Autodesk Fusion 360 part; units mm, degrees
(part 2 of 2)
sketch "Sketch43" plane through (0, 10, 0) normal (0, 1, 0) x (-1, 0, 0)
  line L0 (-47.7, 203) -> (-47.7, 218)
  line L1 (-47.7, 218) -> (-127.2, 218)
  line L2 (-127.2, 218) -> (-127.2, -25)
  line L3 (-127.2, -25) -> (-46.7, -25)
  line L4 (-46.7, -25) -> (-46.7, -10)
  line L5 (-46.7, -10) -> (15, -10)
  line L6 (15, -10) -> (15, -15)
  line L7 (15, -15) -> (30, -15)
  line L8 (30, -15) -> (30, 198)
  line L9 (30, 198) -> (17.475, 208)
  line L10 (17.475, 208) -> (15, 208)
  line L11 (15, 208) -> (15, 203)
  line L12 (15, 203) -> (-47.7, 203)
  circle A0 centre (-63.325, 91) radius 4
  circle A1 centre (-105.075, 102) radius 4
  line L13 (15, 208) -> (30, 208)
  line L14 (30, 208) -> (30, 203)
  line L15 (30, 203) -> (15, 203)
  line L16 (15, 203) -> (15, 208)
  line L17 (30, 203) -> (-47.7, 203)
  line L18 (-47.7, 203) -> (-47.7, 198)
  line L19 (-47.7, 198) -> (30, 198)
  line L20 (30, 198) -> (30, 203)
  line L21 (30, -15) -> (15, -15)
  line L22 (15, -15) -> (15, -10)
  line L23 (15, -10) -> (30, -10)
  line L24 (30, -10) -> (30, -15)
  line L25 (-46.7, -10) -> (30, -10)
  line L26 (30, -10) -> (30, -5)
  line L27 (30, -5) -> (-46.7, -5)
  line L28 (-46.7, -5) -> (-46.7, -10)
  line L29 (15, -10) -> (-46.7, -10)
  line L30 (-46.7, -10) -> (-46.7, -5)
  line L31 (-46.7, -5) -> (15, -5)
  line L32 (15, -5) -> (15, -10)
  dimension "d251" = 15
  dimension "d252" = 5
  dimension "d253" = 5
  dimension "d254" = 15
  dimension "d255" = 5
  dimension "d256" = 5
  constraint horizontal L13
  constraint vertical L14
  constraint horizontal L15
  constraint vertical L16
  constraint coincident L10.end L11.start
  constraint horizontal L17
  constraint vertical L18
  constraint horizontal L19
  constraint vertical L20
  constraint horizontal L21
  constraint vertical L22
  constraint horizontal L23
  constraint vertical L24
  constraint coincident L7.end L8.start
  constraint horizontal L25
  constraint vertical L26
  constraint horizontal L27
  constraint vertical L28
  constraint coincident L4.end L5.start
  constraint horizontal L29
  constraint vertical L30
  constraint horizontal L31
  constraint vertical L32
  measures "d251" distance of L10.end L13.end
  measures "d252" distance of L10.end L11.end
  measures "d253" distance of L14.end L8.end
  measures "d254" distance of L7.end L6.end
  measures "d255" distance of L7.end L23.end
  measures "d256" distance of L4.end L27.end
extrude "Extrude87" cut sketch "Sketch43" against normal blind 5 contours L5 L25 L27 L28 L29 L30 L31 L32 bodies 1
extrude "Extrude88" cut 1 faces at (-25, 8.3333, -15) along direction (0, 0, 1) blind 5 on bodies 1 bodies 1
sketch "Sketch44" plane through (0, 10, 0) normal (0, 1, 0) x (-1, 0, 0)
  line L0 (15, -10) -> (30, -10)
  line L1 (30, -10) -> (30, 198)
  line L2 (30, 198) -> (17.475, 208)
  line L3 (17.475, 208) -> (15, 208)
  line L4 (15, 208) -> (15, 203)
  line L5 (15, 203) -> (-47.7, 203)
  line L6 (-47.7, 203) -> (-47.7, 218)
  line L7 (-47.7, 218) -> (-127.2, 218)
  line L8 (-127.2, 218) -> (-127.2, -25)
  line L9 (-127.2, -25) -> (-46.7, -25)
  line L10 (-46.7, -25) -> (-46.7, -5)
  line L11 (-46.7, -5) -> (15, -5)
  line L12 (15, -5) -> (15, -10)
  circle A0 centre (-63.325, 91) radius 4
  circle A1 centre (-105.075, 102) radius 4
  line L13 (15, 208) -> (30, 208)
  line L14 (30, 208) -> (30, 198)
  line L15 (30, 198) -> (15, 198)
  line L16 (15, 198) -> (15, 208)
  line L17 (15, 203) -> (30, 203)
  line L18 (30, 203) -> (30, 198)
  line L19 (30, 198) -> (15, 198)
  line L20 (15, 198) -> (15, 203)
  line L21 (17.475, 208) -> (30, 198)
  constraint horizontal L13
  constraint vertical L14
  constraint horizontal L15
  constraint vertical L16
  constraint coincident L1.end L2.start
  constraint coincident L3.end L4.start
  constraint horizontal L17
  constraint vertical L18
  constraint horizontal L19
  constraint vertical L20
  constraint coincident L4.end L5.start
  constraint coincident L2.end L3.start
extrude "Extrude89" cut 1 faces at (5.9, 8.3333, 203) along direction (0, 0, -1) blind 5 on bodies 1 bodies 1
sketch "Sketch45" plane through (0, 10, 0) normal (0, 1, 0) x (-1, 0, 0)
  line L0 (30, 198) -> (15, 198)
  line L1 (17.475, 208) -> (17.475, 198)
  line L2 (30, 198) -> (15, 198)
  line L3 (15, 198) -> (15, 193)
  line L4 (15, 193) -> (30, 193)
  line L5 (30, 193) -> (30, 198)
  line L6 (17.475, 203) -> (30, 193)
  point P0 (17.475, 208)
  dimension "d263" = 5
  constraint coincident P0 L1.start
  constraint coincident L0 L1.end
  constraint perpendicular L0 L1
  constraint horizontal L2
  constraint vertical L3
  constraint horizontal L4
  constraint vertical L5
  constraint coincident L0.start L2.start
  constraint midpoint L1 L6.start
  measures "d263" distance of L0.start L4.end
extrude "Extrude90" cut sketch "Sketch44" sketch "Sketch45" against normal blind 5 contours L2 L3 L4 L13 L16 L17 L21 of sketch 2 contours L0 L2 L5 L6 bodies 1
sketch "Sketch46" plane through (0, 10, 0) normal (0, 1, 0) x (-1, 0, 0)
  line L0 (23.7375, 203) -> (15, 203)
  line L1 (15, 203) -> (15, 198)
  line L2 (15, 198) -> (-47.7, 198)
  line L3 (-47.7, 198) -> (-47.7, 218)
  line L4 (-47.7, 218) -> (-127.2, 218)
  line L5 (-127.2, 218) -> (-127.2, -25)
  line L6 (-127.2, -25) -> (-46.7, -25)
  line L7 (-46.7, -25) -> (-46.7, -5)
  line L8 (-46.7, -5) -> (15, -5)
  line L9 (15, -5) -> (15, -10)
  line L10 (15, -10) -> (30, -10)
  line L11 (30, -10) -> (30, 193)
  line L12 (30, 193) -> (23.7375, 198)
  line L13 (23.7375, 198) -> (30, 198)
  line L14 (30, 198) -> (23.7375, 203)
  circle A0 centre (-105.075, 102) radius 4
  circle A1 centre (-63.325, 91) radius 4
  line L15 (15, 203) -> (17.475, 203)
  line L16 (17.475, 203) -> (17.475, 198)
  line L17 (17.475, 198) -> (15, 198)
  line L18 (15, 198) -> (15, 203)
  line L19 (23.7375, 198) -> (17.475, 203)
  dimension "d266" = 2.475
  constraint horizontal L15
  constraint vertical L16
  constraint horizontal L17
  constraint vertical L18
  constraint coincident L0.end L1.start
  constraint coincident L12.end L13.start
  measures "d266" distance of L0.end L15.end
extrude "Extrude91" cut sketch "Sketch46" against normal blind 5 contours L0 L13 L14 L19 bodies 1
sketch "Sketch47" plane through (0, 10, 0) normal (0, 1, 0) x (-1, 0, 0)
  line L0 (30, 193) -> (17.475, 203)
  line L1 (17.475, 203) -> (15, 203)
  line L2 (15, 203) -> (15, 198)
  line L3 (15, 198) -> (-47.7, 198)
  line L4 (-47.7, 198) -> (-47.7, 218)
  line L5 (-47.7, 218) -> (-127.2, 218)
  line L6 (-127.2, 218) -> (-127.2, -25)
  line L7 (-127.2, -25) -> (-46.7, -25)
  line L8 (-46.7, -25) -> (-46.7, -5)
  line L9 (-46.7, -5) -> (15, -5)
  line L10 (15, -5) -> (15, -10)
  line L11 (15, -10) -> (30, -10)
  line L12 (30, -10) -> (30, 193)
  circle A0 centre (-105.075, 102) radius 4
  circle A1 centre (-63.325, 91) radius 4
  line L13 (30, -10) -> (15, -10)
  line L14 (15, -10) -> (15, 13.5)
  line L15 (15, 13.5) -> (30, 13.5)
  line L16 (30, 13.5) -> (30, -10)
  line L17 (30, 13.5) -> (30, 193)
  line L18 (30, 193, 0) -> (30, 193, -5)
  line L19 (30, 193, -5) -> (30, 13.5, -5)
  line L20 (30, 13.5, -5) -> (30, 13.5, 0)
  point P0 (30, 193)
  dimension "d269" = 23.5
  constraint horizontal L13
  constraint vertical L14
  constraint horizontal L15
  constraint vertical L16
  constraint coincident L11.end L12.start
  constraint vertical L17
  constraint coincident P0 L0.start
  measures "d269" distance of L11.end L15.end
extrude "Extrude92" add sketch "Sketch47" along normal blind 10 contours L12 L17 L18 L19 L20 in plane through (-30, 10, 0) normal (-1, 0, 0) bodies 1
sketch "Sketch48" plane through (0, 0, 0) normal (0, 0, 1) x (1, 0, 0)
  point P0 (-15, 10)
extrude "Extrude93" add 1 faces at (-15, 8.3333, 201.3333) along direction (1, 0, 0) blind 62.7 on bodies 1 bodies 1
sketch "Sketch49" plane through (46.7, 0, 0) normal (-1, 0, 0) x (0, 0, 1)
  line L0 (-5, 10) -> (-25, 10)
  line L1 (-25, 10) -> (-25, -20)
  line L2 (-25, -20) -> (-5.4, -20)
  line L3 (-5.4, -20) -> (-5.4, 0)
  line L4 (-5.4, 0) -> (-5, 0)
  line L5 (-5, 0) -> (-5, 10)
  line L6 (-5, 10) -> (-25, 10)
  line L7 (-25, 10) -> (-25, 0)
  line L8 (-25, 0) -> (-5, 0)
  line L9 (-5, 0) -> (-5, 10)
  line L10 (-5, 10) -> (-17.5, 10)
  line L11 (-17.5, 10) -> (-17.5, 0)
  line L12 (-17.5, 0) -> (-5, 0)
  line L13 (-5, 0) -> (-5, 10)
  line L14 (-17.5, 10) -> (-25, 0)
  dimension "d274" = 20
  dimension "d275" = 10
  dimension "d276" = 12.5
  constraint horizontal L6
  constraint vertical L7
  constraint horizontal L8
  constraint vertical L9
  constraint coincident L0.start L5.end
  constraint horizontal L10
  constraint vertical L11
  constraint horizontal L12
  constraint vertical L13
  measures "d274" distance of L0.start L0.end
  measures "d275" distance of L0.start L4.end
  measures "d276" distance of L0.start L10.end
extrude "Extrude94" cut sketch "Sketch49" against normal blind 85 contours L0 L1 L6 L7 L14 bodies 1
sketch "Sketch50" plane through (47.7, 0, 0) normal (-1, 0, 0) x (0, 0, 1)
  line L0 (203, 10) -> (203, 5)
  line L1 (203, 5) -> (198, 5)
  line L2 (198, 5) -> (198, 0)
  line L3 (198, 0) -> (198.4, 0)
  line L4 (198.4, 0) -> (198.4, -20)
  line L5 (198.4, -20) -> (218, -20)
  line L6 (218, -20) -> (218, 10)
  line L7 (218, 10) -> (203, 10)
  line L8 (218, -20) -> (198.4, -20)
  line L9 (198.4, -20) -> (198.4, 0)
  line L10 (198.4, 0) -> (218, 0)
  line L11 (218, 0) -> (218, -20)
  line L12 (198.4, 0) -> (210.9, 0)
  line L13 (210.9, 0) -> (210.9, 10)
  line L14 (210.9, 10) -> (198.4, 10)
  line L15 (198.4, 10) -> (198.4, 0)
  line L16 (210.9, 10) -> (218, 0)
  dimension "d279" = 20
  dimension "d280" = 12.5
  constraint horizontal L8
  constraint vertical L9
  constraint horizontal L10
  constraint vertical L11
  constraint coincident L5.end L6.start
  constraint horizontal L12
  constraint vertical L13
  constraint horizontal L14
  constraint vertical L15
  constraint coincident L3.end L4.start
  measures "d279" distance of L5.end L10.end
  measures "d280" distance of L3.end L12.end
extrude "Extrude95" cut sketch "Sketch50" against normal blind 100 contours L6 L7 L16 bodies 1
extrude "Extrude96" add 1 faces at (-15, 8.3333, -8.3333) along direction (1, 0, 0) blind 61.7 on bodies 1 bodies 1
sketch "Sketch51" plane through (0, 5, 0) normal (0, -1, 0) x (1, 0, 0)
  line L0 (-17.475, 203) -> (-30, 193)
  line L1 (-30, 193) -> (-40, 193)
  line L2 (-40, 193) -> (-40, 13.5)
  line L3 (-40, 13.5) -> (-30, 13.5)
  line L4 (-30, 13.5) -> (-30, -10)
  line L5 (-30, -10) -> (46.7, -10)
  line L6 (46.7, -10) -> (46.7, -5)
  line L7 (46.7, -5) -> (-15, -5)
  line L8 (-15, -5) -> (-15, 198)
  line L9 (-15, 198) -> (47.7, 198)
  line L10 (47.7, 198) -> (47.7, 203)
  line L11 (47.7, 203) -> (-17.475, 203)
  line L12 (-40, 13.5) -> (-30.25, 13.5)
  line L13 (-30.25, 13.5) -> (-30.25, 193)
  line L14 (-30.25, 193) -> (-40, 193)
  line L15 (-40, 193) -> (-40, 13.5)
  dimension "d285" = 9.75
  constraint horizontal L12
  constraint vertical L13
  constraint horizontal L14
  constraint vertical L15
  constraint coincident L2.end L3.start
  measures "d285" distance of L2.end L12.end
extrude "Extrude97" add sketch "Sketch51" along normal blind 15 contours L1 L2 L3 L12 L13 L14 L15 bodies 1
extrude "Extrude98" add 1 faces at (-0.2101, 10, 99.3654) along direction (0, 1, 0) blind 5 on bodies 1 bodies 1
extrude "Extrude99" cut 1 faces at (-36.75, -10, 133.1667) along direction (0, 1, 0) blind 15 on bodies 1 bodies 1
sketch "Sketch52" plane through (0, -20, 0) normal (0, -1, 0) x (1, 0, 0)
  line L0 (47.7, 218) -> (47.7, 198.4)
  line L1 (47.7, 198.4) -> (122.2, 198.4)
  line L2 (122.2, 198.4) -> (127.2, 198.4)
  line L3 (127.2, 198.4) -> (127.2, 218)
  line L4 (127.2, 218) -> (47.7, 218)
  line L5 (127.2, 218) -> (120.2, 218)
  line L6 (120.2, 218) -> (120.2, 211)
  line L7 (120.2, 211) -> (127.2, 211)
  line L8 (127.2, 211) -> (127.2, 218)
  line L9 (127.2, 211) -> (120.2, 218)
  dimension "d292" = 7
  dimension "d293" = 7
  constraint horizontal L5
  constraint vertical L6
  constraint horizontal L7
  constraint vertical L8
  constraint coincident L3.end L4.start
  measures "d292" distance of L3.end L5.end
  measures "d293" distance of L3.end L7.end
extrude "Extrude100" cut sketch "Sketch52" against normal blind 40 contours L3 L4 L5 L8 L9 bodies 1
sketch "Sketch53" plane through (0, -20, 0) normal (0, -1, 0) x (1, 0, 0)
  line L0 (46.7, -25) -> (127.2, -25)
  line L1 (127.2, -25) -> (127.2, -5.4)
  line L2 (127.2, -5.4) -> (122.2, -5.4)
  line L3 (122.2, -5.4) -> (46.7, -5.4)
  line L4 (46.7, -5.4) -> (46.7, -25)
  line L5 (127.2, -25) -> (120.2, -25)
  line L6 (120.2, -25) -> (120.2, -18)
  line L7 (120.2, -18) -> (127.2, -18)
  line L8 (127.2, -18) -> (127.2, -25)
  line L9 (127.2, -18) -> (120.2, -25)
  dimension "d296" = 7
  dimension "d297" = 7
  constraint horizontal L5
  constraint vertical L6
  constraint horizontal L7
  constraint vertical L8
  constraint coincident L0.end L1.start
  measures "d296" distance of L0.end L5.end
  measures "d297" distance of L0.end L7.end
extrude "Extrude101" cut sketch "Sketch53" against normal blind 40 contours L0 L1 L5 L8 L9 bodies 1
sketch "Sketch54" plane through (0, 0, 210.9) normal (0, 0, 1) x (1, 0, 0)
  line L0 (47.7, 10) -> (127.2, 10)
  line L1 (127.2, 10) -> (127.2, 15)
  line L2 (127.2, 15) -> (47.7, 15)
  line L3 (47.7, 15) -> (47.7, 10)
  line L4 (127.2, 15) -> (122.2, 15)
  line L5 (122.2, 15) -> (122.2, 10)
  line L6 (122.2, 10) -> (127.2, 10)
  line L7 (127.2, 10) -> (127.2, 15)
  line L8 (127.2, 10) -> (122.2, 15)
  dimension "d300" = 5
  constraint horizontal L4
  constraint vertical L5
  constraint horizontal L6
  constraint vertical L7
  constraint coincident L1.end L2.start
  constraint coincident L0.end L1.start
  measures "d300" distance of L1.end L4.end
extrude "Extrude102" cut sketch "Sketch54" against normal blind 360 contours L1 L2 L4 L7 L8 bodies 1
sketch "Sketch55" plane through (46.7, 0, 0) normal (-1, 0, 0) x (0, 0, 1)
  line L0 (-10, 5) -> (-10, 15)
  line L1 (-10, 15) -> (-17.5, 15)
  line L2 (-17.5, 15) -> (-17.5, 10)
  line L3 (-17.5, 10) -> (-25, 0)
  line L4 (-25, 0) -> (-25, -20)
  line L5 (-25, -20) -> (-5.4, -20)
  line L6 (-5.4, -20) -> (-5.4, 0)
  line L7 (-5.4, 0) -> (-5, 0)
  line L8 (-5, 0) -> (-5, 5)
  line L9 (-5, 5) -> (-10, 5)
  line L10 (-25, -20) -> (-18, -20)
  line L11 (-18, -20) -> (-18, -13)
  line L12 (-18, -13) -> (-25, -13)
  line L13 (-25, -13) -> (-25, -20)
  line L14 (218, -20, -1) -> (211, -20, -1)
  line L15 (211, -20, -1) -> (211, -13, -1)
  line L16 (211, -13, -1) -> (218, -13, -1)
  line L17 (218, -13, -1) -> (218, -20, -1)
  line L18 (-25, -13) -> (-18, -20)
  line L19 (218, -13, -1) -> (211, -20, -1)
  point P0 (218, -20)
  dimension "d303" = 7
  dimension "d304" = 7
  dimension "d305" = 7
  dimension "d306" = 7
  constraint horizontal L10
  constraint vertical L11
  constraint horizontal L12
  constraint vertical L13
  constraint coincident L4.end L5.start
  measures "d303" distance of L4.end L10.end
  measures "d304" distance of L4.end L12.end
extrude "Extrude103" cut sketch "Sketch55" against normal blind 140 contours L4 L5 L10 L13 L18 bodies 1
sketch "Sketch56" plane through (47.7, 0, 0) normal (-1, 0, 0) x (0, 0, 1)
  line L0 (218, 0) -> (210.9, 10)
  line L1 (210.9, 10) -> (210.9, 15)
  line L2 (210.9, 15) -> (203, 15)
  line L3 (203, 15) -> (203, 5)
  line L4 (203, 5) -> (198, 5)
  line L5 (198, 5) -> (198, 0)
  line L6 (198, 0) -> (198.4, 0)
  line L7 (198.4, 0) -> (198.4, -20)
  line L8 (198.4, -20) -> (218, -20)
  line L9 (218, -20) -> (218, 0)
  line L10 (218, -20) -> (211, -20)
  line L11 (211, -20) -> (211, -13)
  line L12 (211, -13) -> (218, -13)
  line L13 (218, -13) -> (218, -20)
  line L14 (211, -20) -> (218, -13)
  dimension "d309" = 7
  dimension "d310" = 7
  constraint horizontal L10
  constraint vertical L11
  constraint horizontal L12
  constraint vertical L13
  constraint coincident L8.end L9.start
  measures "d309" distance of L8.end L10.end
  measures "d310" distance of L8.end L12.end
extrude "Extrude104" cut sketch "Sketch56" against normal blind 110 contours L8 L9 L10 L13 L14 bodies 1
sketch "Sketch57" plane through (47.7, 0, 0) normal (-1, 0, 0) x (0, 0, 1)
  line L0 (211, -20) -> (218, -13)
  line L1 (218, -13) -> (218, 0)
  line L2 (218, 0) -> (210.9, 10)
  line L3 (210.9, 10) -> (210.9, 15)
  line L4 (210.9, 15) -> (203, 15)
  line L5 (203, 15) -> (203, 5)
  line L6 (203, 5) -> (198, 5)
  line L7 (198, 5) -> (198, 0)
  line L8 (198, 0) -> (198.4, 0)
  line L9 (198.4, 0) -> (198.4, -20)
  line L10 (198.4, -20) -> (211, -20)
  line L11 (203, 15) -> (208, 15)
  line L12 (208, 15) -> (208, 10)
  line L13 (208, 10) -> (203, 10)
  line L14 (203, 10) -> (203, 15)
  line L15 (208, 10) -> (210.9, 10)
  line L16 (210.9, 10) -> (210.9, 15)
  line L17 (210.9, 15) -> (208, 15)
  line L18 (208, 15) -> (208, 10)
  line L19 (203, 15) -> (208, 10)
  dimension "d313" = 5
  dimension "d314" = 5
  constraint horizontal L11
  constraint vertical L12
  constraint horizontal L13
  constraint vertical L14
  constraint coincident L4.end L5.start
  constraint horizontal L15
  constraint vertical L16
  constraint horizontal L17
  constraint vertical L18
  constraint coincident L3.end L4.start
  measures "d313" distance of L4.end L11.end
  measures "d314" distance of L4.end L13.end
extrude "Extrude105" cut sketch "Sketch57" against normal blind 82 contours L3 L4 L12 L15 L16 L17 L18 | L4 L11 L12 L18 L19 bodies 1
sketch "Sketch58" plane through (46.7, 0, 0) normal (-1, 0, 0) x (0, 0, 1)
  line L0 (-25, -13) -> (-18, -20)
  line L1 (-18, -20) -> (-5.4, -20)
  line L2 (-5.4, -20) -> (-5.4, 0)
  line L3 (-5.4, 0) -> (-5, 0)
  line L4 (-5, 0) -> (-5, 5)
  line L5 (-5, 5) -> (-10, 5)
  line L6 (-10, 5) -> (-10, 15)
  line L7 (-10, 15) -> (-17.5, 15)
  line L8 (-17.5, 15) -> (-17.5, 10)
  line L9 (-17.5, 10) -> (-25, 0)
  line L10 (-25, 0) -> (-25, -13)
  line L11 (-10, 15) -> (-15, 15)
  line L12 (-15, 15) -> (-15, 10)
  line L13 (-15, 10) -> (-10, 10)
  line L14 (-10, 10) -> (-10, 15)
  line L15 (-17.5, 15) -> (-15, 15)
  line L16 (-15, 15) -> (-15, 10)
  line L17 (-15, 10) -> (-17.5, 10)
  line L18 (-17.5, 10) -> (-17.5, 15)
  line L19 (-15, 10) -> (-10, 15)
  dimension "d317" = 5
  constraint horizontal L11
  constraint vertical L12
  constraint horizontal L13
  constraint vertical L14
  constraint coincident L6.end L7.start
  constraint horizontal L15
  constraint vertical L16
  constraint horizontal L17
  constraint vertical L18
  constraint coincident L7.end L8.start
  measures "d317" distance of L6.end L11.end
extrude "Extrude106" cut sketch "Sketch58" against normal blind 103 contours L7 L8 L12 L15 L16 L17 L18 | L7 L11 L12 L16 L19 bodies 1
sketch "Sketch59" plane through (46.7, 0, 0) normal (-1, 0, 0) x (0, 0, 1)
  line L0 (-15, 10) -> (-17.5, 10)
  line L1 (-17.5, 10) -> (-25, 0)
  line L2 (-25, 0) -> (-25, -13)
  line L3 (-25, -13) -> (-18, -20)
  line L4 (-18, -20) -> (-5.4, -20)
  line L5 (-5.4, -20) -> (-5.4, 0)
  line L6 (-5.4, 0) -> (-5, 0)
  line L7 (-5, 0) -> (-5, 5)
  line L8 (-5, 5) -> (-10, 5)
  line L9 (-10, 5) -> (-10, 15)
  line L10 (-10, 15) -> (-15, 10)
  line L11 (-5, 5) -> (-21.25, 5)
  line L12 (-25, -13) -> (-5.4, -13)
  line L13 (-5.4, -13) -> (-5.4, -20)
  line L14 (-5.4, -20) -> (-25, -20)
  line L15 (-25, -20) -> (-25, -13)
  constraint coincident L7.end L8.start
  constraint midpoint L1 L11.end
  constraint horizontal L12
  constraint vertical L13
  constraint horizontal L14
  constraint vertical L15
  constraint coincident L4.end L5.start
  constraint coincident L2.end L3.start
extrude "Extrude107" cut sketch "Sketch59" against normal blind 75 contours L3 L4 L5 L12 L13 L14 bodies 1
sketch "Sketch60" plane through (47.7, 0, 0) normal (-1, 0, 0) x (0, 0, 1)
  line L0 (208, 10) -> (203, 15)
  line L1 (203, 15) -> (203, 5)
  line L2 (203, 5) -> (198, 5)
  line L3 (198, 5) -> (198, 0)
  line L4 (198, 0) -> (198.4, 0)
  line L5 (198.4, 0) -> (198.4, -20)
  line L6 (198.4, -20) -> (211, -20)
  line L7 (211, -20) -> (218, -13)
  line L8 (218, -13) -> (218, 0)
  line L9 (218, 0) -> (210.9, 10)
  line L10 (210.9, 10) -> (208, 10)
  line L11 (218, -13) -> (198.4, -13)
  line L12 (198.4, -13) -> (198.4, -20)
  line L13 (198.4, -20) -> (218, -20)
  line L14 (218, -20) -> (218, -13)
  constraint horizontal L11
  constraint vertical L12
  constraint horizontal L13
  constraint vertical L14
  constraint coincident L5.end L6.start
  constraint coincident L7.end L8.start
extrude "Extrude108" cut sketch "Sketch60" against normal blind 74.5 contours L5 L6 L7 L11 L12 L13 bodies 1
sketch "Sketch61" plane through (0, 0, 0) normal (0, -1, 0) x (1, 0, 0)
  line L0 (47.7, 198) -> (-15, 198)
  line L1 (-15, 198) -> (-15, -5)
  line L2 (-15, -5) -> (46.7, -5)
  line L3 (46.7, -5) -> (46.7, -5.4)
  line L4 (46.7, -5.4) -> (122.2, -5.4)
  line L5 (122.2, -5.4) -> (122.2, 0)
  line L6 (122.2, 0) -> (112.7, 0)
  line L7 (112.7, 0) -> (112.7, 193)
  line L8 (112.7, 193) -> (122.2, 193)
  line L9 (122.2, 193) -> (122.2, 198.4)
  line L10 (122.2, 198.4) -> (47.7, 198.4)
  line L11 (47.7, 198.4) -> (47.7, 198)
  circle A0 centre (63.325, 91) radius 4
  circle A1 centre (105.075, 102) radius 4
  circle A2 centre (105.075, 102) radius 4
  circle A3 centre (63.325, 91) radius 4
  circle A4 through (109.075, 102, -15) (103.075, 105.4641, -15) (103.075, 98.5359, -15)
  circle A5 through (109.075, 102, -15) (103.075, 105.4641, -15) (103.075, 98.5359, -15)
  circle A6 through (67.325, 91, -15) (61.325, 94.4641, -15) (61.325, 87.5359, -15)
  circle A7 through (67.325, 91, -15) (61.325, 94.4641, -15) (61.325, 87.5359, -15)
  line L12 (105.075, 102, -15) -> (63.325, 102, -15)
  line L13 (63.325, 102, -15) -> (63.325, 91, -15)
  line L14 (63.325, 91, -15) -> (105.075, 91, -15)
  line L15 (105.075, 91, -15) -> (105.075, 102, -15)
  constraint concentric A1 A2
  constraint concentric A0 A3
  constraint coincident A0.centre A3.centre
  constraint coincident A1.centre A2.centre
extrude "Extrude109" add sketch "Sketch61" along normal blind 15 contours A4 A5 L12 L15 | A4 A5 L12 L15 | A6 A7 L13 L14 | A6 A7 L13 L14 in plane through (0, 15, 0) normal (0, -1, 0) bodies 1
sketch "Sketch62" plane through (0, 15, 0) normal (0, 1, 0) x (-1, 0, 0)
  line L0 (-122.2, -10) -> (-46.7, -10)
  line L1 (-46.7, -10) -> (30, -10)
  line L2 (30, -10) -> (30, 13.5)
  line L3 (30, 13.5) -> (40, 13.5)
  line L4 (40, 13.5) -> (40, 193)
  line L5 (40, 193) -> (30, 193)
  line L6 (30, 193) -> (17.475, 203)
  line L7 (17.475, 203) -> (-47.7, 203)
  line L8 (-47.7, 203) -> (-122.2, 203)
  line L9 (-122.2, 203) -> (-122.2, -10)
  line L10 (-122.2, 203) -> (-100.075, 203)
  line L11 (-100.075, 203) -> (-100.075, 102)
  line L12 (-100.075, 102) -> (-122.2, 102)
  line L13 (-122.2, 102) -> (-122.2, 203)
  line L14 (-100.075, 102) -> (-58.325, 102)
  line L15 (-58.325, 102) -> (-58.325, 91)
  line L16 (-58.325, 91) -> (-100.075, 91)
  line L17 (-100.075, 91) -> (-100.075, 102)
  circle A0 centre (-100.075, 102) radius 4
  circle A1 centre (-58.325, 91) radius 4
  dimension "d326" = 22.125
  dimension "d327" = 101
  dimension "d328" = 41.75
  dimension "d329" = 11
  dimension "d330" = 8
  dimension "d331" = 8
  constraint horizontal L10
  constraint vertical L11
  constraint horizontal L12
  constraint vertical L13
  constraint coincident L8.end L9.start
  constraint horizontal L14
  constraint vertical L15
  constraint horizontal L16
  constraint vertical L17
  constraint coincident L11.end L12.start
  constraint coincident L15.end L16.start
  measures "d326" distance of L8.end L10.end
  measures "d327" distance of L8.end L12.end
  measures "d328" distance of L11.end L14.end
  measures "d329" distance of L11.end L16.end
  measures "d330" diameter of A0
  measures "d331" diameter of A1
extrude "Extrude110" cut sketch "Sketch62" against normal blind 15 contours L11 L12 A0 | L12 L17 A0 | L11 L14 A0 | L14 L17 A0 | L15 L16 A1 | L15 L16 A1 bodies 1
sketch "Sketch63" plane through (0, 15, 0) normal (0, 1, 0) x (-1, 0, 0)
  circle A0 centre (-100.075, 102) radius 4
  line L0 (-122.2, -10) -> (-46.7, -10)
  line L1 (-46.7, -10) -> (30, -10)
  line L2 (30, -10) -> (30, 13.5)
  line L3 (30, 13.5) -> (40, 13.5)
  line L4 (40, 13.5) -> (40, 193)
  line L5 (40, 193) -> (30, 193)
  line L6 (30, 193) -> (17.475, 203)
  line L7 (17.475, 203) -> (-47.7, 203)
  line L8 (-47.7, 203) -> (-122.2, 203)
  line L9 (-122.2, 203) -> (-122.2, -10)
  circle A1 through (-96.075, 102, -15) (-102.075, 105.4641, -15) (-102.075, 98.5359, -15)
  circle A2 through (-96.075, 102, -15) (-102.075, 105.4641, -15) (-102.075, 98.5359, -15)
  circle A3 through (-54.325, 91, -15) (-60.325, 94.4641, -15) (-60.325, 87.5359, -15)
  circle A4 through (-54.325, 91, -15) (-60.325, 94.4641, -15) (-60.325, 87.5359, -15)
  line L10 (-127.2, 198.4, -318) -> (-122.2, 198.4, -318)
  line L11 (-122.2, 198.4, -318) -> (-122.2, -5.4, -318)
  line L12 (-122.2, -5.4, -318) -> (-127.2, -5.4, -318)
  line L13 (-127.2, -5.4, -318) -> (-127.2, 198.4, -318)
  point P0 (-127.2, 198.4)
  point P1 (-122.2, -5.4)
extrude "Extrude111" add sketch "Sketch63" against normal blind 20 contours L10 L11 L12 L13 in plane through (0, -303, 0) normal (0, 1, 0) bodies 1
sketch "Sketch64" plane through (0, -323, 0) normal (0, -1, 0) x (1, 0, 0)
  line L0 (122.2, -5.4) -> (127.2, -5.4)
  line L1 (127.2, -5.4) -> (127.2, 198.4)
  line L2 (127.2, 198.4) -> (122.2, 198.4)
  line L3 (122.2, 198.4) -> (122.2, -5.4)
  line L4 (127.2, 198.4) -> (122.2, 198.4)
  line L5 (122.2, 198.4) -> (122.2, 193.4)
  line L6 (122.2, 193.4) -> (127.2, 193.4)
  line L7 (127.2, 193.4) -> (127.2, 198.4)
  line L8 (127.2, -5.4) -> (122.2, -5.4)
  line L9 (122.2, -5.4) -> (122.2, -0.4)
  line L10 (122.2, -0.4) -> (127.2, -0.4)
  line L11 (127.2, -0.4) -> (127.2, -5.4)
  line L12 (127.2, 193.4) -> (122.2, 198.4)
  line L13 (127.2, -0.4) -> (122.2, -5.4)
  dimension "d336" = 5
  dimension "d337" = 5
  dimension "d338" = 5
  constraint horizontal L4
  constraint vertical L5
  constraint horizontal L6
  constraint vertical L7
  constraint coincident L1.end L2.start
  constraint horizontal L8
  constraint vertical L9
  constraint horizontal L10
  constraint vertical L11
  constraint coincident L0.end L1.start
  constraint coincident L2.end L3.start
  constraint coincident L0.start L3.end
  measures "d336" distance of L1.end L6.end
  measures "d337" distance of L0.end L0.start
  measures "d338" distance of L0.end L10.end
extrude "Extrude112" cut sketch "Sketch64" against normal blind 303 contours L0 L1 L8 L11 L13 | L1 L2 L4 L7 L12 bodies 1
sketch "Sketch65" plane through (0, 0, 13.5) normal (0, 0, -1) x (-1, 0, 0)
  line L0 (30, 5) -> (40, 5)
  line L1 (40, 5) -> (40, 15)
  line L2 (40, 15) -> (30, 15)
  line L3 (30, 15) -> (30, 5)
  line L4 (40, 15) -> (35, 15)
  line L5 (35, 15) -> (35, 10)
  line L6 (35, 10) -> (40, 10)
  line L7 (40, 10) -> (40, 15)
  line L8 (40, 10) -> (35, 15)
  dimension "d341" = 5
  dimension "d342" = 5
  constraint horizontal L4
  constraint vertical L5
  constraint horizontal L6
  constraint vertical L7
  constraint coincident L1.end L2.start
  measures "d341" distance of L1.end L4.end
  measures "d342" distance of L1.end L6.end
extrude "Extrude113" cut sketch "Sketch65" against normal blind 220 contours L1 L2 L4 L7 L8 bodies 1
sketch "Sketch66" plane through (0, 15, 0) normal (0, 1, 0) x (-1, 0, 0)
  line L0 (35, 13.5) -> (35, 193)
  line L1 (35, 193) -> (30, 193)
  line L2 (30, 193) -> (17.475, 203)
  line L3 (17.475, 203) -> (-47.7, 203)
  line L4 (-47.7, 203) -> (-122.2, 203)
  line L5 (-122.2, 203) -> (-122.2, -10)
  line L6 (-122.2, -10) -> (-46.7, -10)
  line L7 (-46.7, -10) -> (30, -10)
  line L8 (30, -10) -> (30, 13.5)
  line L9 (30, 13.5) -> (35, 13.5)
  circle A0 centre (-58.325, 91) radius 4
  circle A1 centre (-100.075, 102) radius 4
  circle A2 centre (-100.075, 102) radius 4
  circle A3 centre (-58.325, 91) radius 4
  circle A4 through (-54.325, 91, -15) (-60.325, 94.4641, -15) (-60.325, 87.5359, -15)
  circle A5 through (-54.325, 91, -15) (-60.325, 94.4641, -15) (-60.325, 87.5359, -15)
  circle A6 through (-96.075, 102, -15) (-102.075, 105.4641, -15) (-102.075, 98.5359, -15)
  circle A7 through (-96.075, 102, -15) (-102.075, 105.4641, -15) (-102.075, 98.5359, -15)
  constraint concentric A1 A2
  constraint concentric A0 A3
